Autodesk Fusion 360 part; units mm, degrees
note: some values were not read from the file. Chosen so that the rebuilt part matches the saved one: which bodies a step acts on; which face or edge a step refers to. Set by a fixed rule: which sketch regions a step uses.
(part 2 of 2)
sketch "Sketch6" plane through (-200.2067, 80.9105, -74.8317) normal (0, 0, 1) x (1, 0, 0) in component "Component''"
  line L0 (-10, -0.5448) -> (10.3529, -0.5448)
  line L1 (10.3529, -0.5448) -> (10.3529, -20)
  line L2 (10.3529, -20) -> (-10, -20)
  line L3 (-10, -20) -> (-10, -0.5448)
  spline S0 degree 5 poles (-10, -20) (-10.0372, -19.5712) (-10.0962, -18.7187) (-10.1386, -17.4552) (-10.1027, -15.7996) (-9.8996, -13.7718) (-9.5308, -11.7785) (-8.9877, -9.8141) (-8.2642, -7.8774) (-7.3627, -5.9724) (-6.2871, -4.1068) (-5.2896, -2.6532) (-4.4647, -1.5886) (-3.8805, -0.8907) (-3.5799, -0.5448) knots 0 0 0 0 0 0 0.1 0.2 0.3 0.4 0.5 0.6 0.7 0.8 0.9 1 1 1 1 1 1
  line L4 (-10, -20) -> (0.1765, -20)
  line L5 (0.1765, -20) -> (0, 0)
  spline S1 degree 5 poles (10.3513, -19.8204) (10.381, -19.3911) (10.4249, -18.5376) (10.445, -17.2736) (10.3799, -15.6189) (10.1411, -13.595) (9.7372, -11.6085) (9.1594, -9.654) (8.4019, -7.7303) (7.4669, -5.8415) (6.3585, -3.9952) (5.3356, -2.5594) (4.4921, -1.5095) (3.8957, -0.8221) (3.5889, -0.4815) knots 0 0 0 0 0 0 0.1 0.2 0.3 0.4 0.5 0.6 0.7 0.8 0.9 1 1 1 1 1 1
  line L6 (-9.8027, -22.275) -> (-10.1973, -17.725)
  line L7 (-5.1045, -2.2991) -> (-2.0553, 1.2095)
  line L8 (10.1942, -22.0986) -> (10.5085, -17.5423)
  line L9 (5.1443, -2.2086) -> (2.0336, 1.2456)
  point P0 (-9, -10)
  point P1 (9.175, -9.8396)
  constraint horizontal L0
  constraint vertical L1
  constraint horizontal L2
  constraint vertical L3
  constraint coincident L0 S0.end
  constraint midpoint L2 L4.end
  constraint coincident L5.end origin
  constraint midpoint L2.end L6
  constraint midpoint S0.end L7
  constraint symmetric L2.end L5 S1.start
  constraint symmetric P0 L5 P1
  constraint symmetric S0.end L5 S1.end
  constraint symmetric L5 L6.start L8.start
  constraint symmetric L5 L6.end L8.end
  constraint symmetric L5 L7.start L9.start
  constraint symmetric L5 L7.end L9.end
ref_plane "WorkPlane2" through (-210.2067, 69.5065, -84.8317) normal (-1, 0, 0) x (0, 0, -1) in component "Component''"
sketch "Sketch7" plane through (-210.2067, 69.5065, -84.8317) normal (-1, 0, 0) x (0, 0, -1) in component "Component''"
  line L0 (10, -10.7188) -> (-10, -10.7188)
  line L1 (-10, -10.7188) -> (-10, 8)
  line L2 (-10, 8) -> (10, 8)
  line L3 (10, 8) -> (10, -10.7188)
  spline S0 degree 5 poles (10, 8) (10, 7.8665) (9.9837, 7.5192) (9.9104, 6.7573) (9.718, 5.2968) (9.3349, 2.936) (8.8272, 0.3007) (8.2129, -2.3455) (7.508, -4.7777) (6.7272, -6.8686) (5.8823, -8.5719) (5.1617, -9.62) (4.5983, -10.235) (4.2126, -10.57) (4.0172, -10.7188) knots 0 0 0 0 0 0 0.1 0.2 0.3 0.4 0.5 0.6 0.7 0.8 0.9 1 1 1 1 1 1
  line L4 (10, 9) -> (10, 7)
  line L5 (10, 8) -> (0, 8)
  line L6 (0, -10.7188) -> (0, 8)
  spline S1 degree 5 poles (-10, 8) (-10, 7.8665) (-9.9837, 7.5192) (-9.9104, 6.7573) (-9.718, 5.2968) (-9.3349, 2.936) (-8.8272, 0.3007) (-8.2129, -2.3455) (-7.508, -4.7777) (-6.7272, -6.8686) (-5.8823, -8.5719) (-5.1617, -9.62) (-4.5983, -10.235) (-4.2126, -10.57) (-4.0172, -10.7188) knots 0 0 0 0 0 0 0.1 0.2 0.3 0.4 0.5 0.6 0.7 0.8 0.9 1 1 1 1 1 1
  line L7 (5.6343, -9.487) -> (2.4001, -11.9507)
  line L8 (-10, 9) -> (-10, 7)
  line L9 (-5.6343, -9.487) -> (-2.4001, -11.9507)
  point P0 (8, -3)
  point P1 (-8, -3)
  constraint horizontal L0
  constraint vertical L1
  constraint horizontal L2
  constraint vertical L3
  constraint coincident L0 S0.end
  constraint midpoint L2.end L4
  constraint coincident L3 L4.end
  constraint midpoint L2 L5.end
  constraint midpoint L0 L6.start
  constraint midpoint S0.end L7
  constraint symmetric L2.end L6 L1.end
  constraint symmetric P0 L6 P1
  constraint symmetric S0.end L6 S1.end
  constraint symmetric L4.start L6 L8.start
  constraint symmetric L4.end L6 L8.end
  constraint symmetric L6 L7.start L9.start
  constraint symmetric L6 L7.end L9.end
extrude "Extrude14" cut sketch "Sketch7" against normal blind 25 contours L0 L3 S0 L4 | L0 L1 S1 L8 bodies 29 in component "Component''"
extrude "Extrude13" cut sketch "Sketch6" against normal blind 43 contours L0 L3 S0 | L0 L1 S1 bodies 29 in component "Component''"
mirror "MirrorComponent1" about plane through (0, 0, 0) normal (0, 0, 1) of bodies 37 36 38 30 31 32 33 34 35 29 39 28 27 makes body 40 at (-199.7772, 30, 65.1742) makes body 41 at (-220.1136, 40.2115, 86.0737) makes body 42 at (-220.0763, 30.2115, 83.0929) makes body 43 at (-232.6638, 27.9703, 102.663) makes body 44 at (-167.7502, 27.9681, 67.0008) makes body 45 at (-200.9929, 27.9703, 121.856) makes body 46 at (-231.8775, 27.9703, 65.6387) makes body 47 at (-199.4204, 27.9703, 47.8074) makes body 48 at (-168.5358, 27.9703, 104.0248) makes body 49 at (-192.4758, 69.7322, 91.1747) makes body 50 at (-210.157, 36.6667, 83.836) makes body 51 at (-200.8838, 56.6667, 82.4252) makes body 52 at (-240.6563, 23.3333, 86.8505) in component "Component3(Mirror)"
mirror "MirrorComponent2" about plane through (0, 0, 0) normal (0, 0, 1) of bodies 51 49 43 44 45 46 47 48 41 40 42 50 52 makes body 53 at (-200.8838, 56.6667, -82.4252) makes body 54 at (-192.4758, 69.7322, -91.1747) makes body 55 at (-232.6638, 27.9703, -102.663) makes body 56 at (-167.7502, 27.9681, -67.0008) makes body 57 at (-200.9929, 27.9703, -121.856) makes body 58 at (-231.8775, 27.9703, -65.6387) makes body 59 at (-199.4204, 27.9703, -47.8074) makes body 60 at (-168.5358, 27.9703, -104.0248) makes body 61 at (-220.1136, 40.2115, -86.0737) makes body 62 at (-199.7772, 30, -65.1742) makes body 63 at (-220.0763, 30.2115, -83.0929) makes body 64 at (-210.157, 36.6667, -83.836) makes body 65 at (-240.6563, 23.3333, -86.8505) in component "Component3(Mirror)(Mirror)"
mirror "MirrorComponent2'" about plane through (0, 0, 0) normal (0, 0, 1) of bodies 37 36 38 30 31 32 33 34 35 29 39 28 27 makes body 66 at (-199.7772, 30, 65.1742) makes body 67 at (-220.1136, 40.2115, 86.0737) makes body 68 at (-220.0763, 30.2115, 83.0929) makes body 69 at (-232.6638, 27.9703, 102.663) makes body 70 at (-167.7502, 27.9681, 67.0008) makes body 71 at (-200.9929, 27.9703, 121.856) makes body 72 at (-231.8775, 27.9703, 65.6387) makes body 73 at (-199.4204, 27.9703, 47.8074) makes body 74 at (-168.5358, 27.9703, 104.0248) makes body 75 at (-192.4758, 69.7322, 91.1747) makes body 76 at (-210.157, 36.6667, 83.836) makes body 77 at (-200.8838, 56.6667, 82.4252) makes body 78 at (-240.6563, 23.3333, 86.8505) in component "Component3(Mirror) (1)"
component "Component" placed x (1, 0, 0) y (0, 1, 0) z (0, 0, 1) at (0, 0, 0)
component "Component'" placed x (1, 0, 0) y (0, 1, 0) z (0, 0, 1) at (0, 0, 0)
component "Component''" placed x (1, 0, 0) y (0, 1, 0) z (0, 0, 1) at (0, 0, 0)
component "Component3(Mirror)" placed x (-1, 0, 0) y (0, 1, 0) z (0, 0, -1) at (0, 0, 0)
component "Component3(Mirror) (1)" placed x (1, 0, 0) y (0, 1, 0) z (0, 0, 1) at (0, 0, 0)
component "Component3(Mirror)(Mirror)" placed x (-1, 0, 0) y (0, 1, 0) z (0, 0, -1) at (0, 0, 0)
